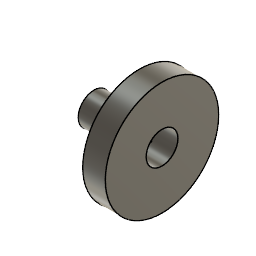
BEYBLADE (Autodesk Fusion 360 design; units mm, degrees)
part number: 2026-01-28-16-23-30-259
Autodesk Fusion 360 part; units mm, degrees
cylinder "CylinderPrimitive1" add diameter 50 height 10 placed x (0, 0, -1) y (0, 1, 0) z (1, 0, 0) at (0, 0, 0) makes body 1
sketch "Sketch2" plane through (0, 0, 0) normal (1, 0, 0) x (0, 1, 0)
cylinder "CylinderPrimitive2" cut diameter 14 height 10 placed x (0, 0, -1) y (0, 1, 0) z (1, 0, 0) at (0, 0, 0) bodies 1
cylinder "CylinderPrimitive3" add diameter 14 height -20 placed x (0, 0, -1) y (0, 1, 0) z (1, 0, 0) at (0, 0, 0) separate body makes body 2
cylinder "CylinderPrimitive4" add diameter 1 height 5 placed x (0, 0, -1) y (0, 1, 0) z (1, 0, 0) at (0, 0, 0) bodies 2
